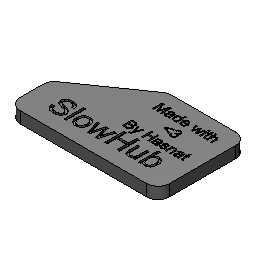
slowhub assembled (Autodesk Fusion 360 archive; units mm, degrees)
design "Slowhub Top"
part number: 2026-06-01-11-18-53-396
Autodesk Fusion 360 part; units mm, degrees
sketch "Sketch1" plane through (0, 0, 0) normal (0, 0, 1) x (1, 0, 0)
  arc A0 through (105.9986, -116.1185, 3) (107.7559, -120.3611, 3) (111.9985, -122.1184, 3)
  arc A1 through (177.7077, -122.1184, 3) (181.9503, -120.3611, 3) (183.7076, -116.1185, 3)
  arc A2 through (183.7076, -81.7289, 3) (181.9503, -77.4863, 3) (177.7077, -75.729, 3)
  arc A3 through (180.7076, -81.7289, 3) (179.829, -79.6076, 3) (177.7077, -78.729, 3)
  arc A4 through (144.4062, -75.729, 3) (142.6026, -76.0065, 3) (140.9659, -76.8133, 3)
  arc A5 through (108.5627, -99.4849, 3) (106.6768, -101.6374, 3) (106.0025, -104.4186, 3)
  arc A6 through (177.7077, -119.1184, 3) (179.829, -118.2398, 3) (180.7076, -116.1185, 3)
  arc A7 through (180.7076, -81.7289, 3) (179.829, -79.6076, 3) (177.7077, -78.729, 3)
  arc A8 through (144.4062, -78.729, 3) (143.5042, -78.8678, 3) (142.6857, -79.2713, 3)
  arc A9 through (110.2827, -101.9429, 3) (109.3377, -103.023, 3) (109.0025, -104.4186, 3)
  arc A10 through (108.9986, -116.1185, 3) (109.8772, -118.2398, 3) (111.9985, -119.1184, 3)
  line L0 (177.7077, -122.1184, 3) -> (111.9985, -122.1184, 3)
  line L1 (183.7076, -81.7289, 3) -> (183.7076, -116.1185, 3)
  line L2 (177.7077, -75.729, 3) -> (144.4062, -75.729, 3)
  line L3 (140.9659, -76.8133, 3) -> (108.5627, -99.4849, 3)
  line L4 (106.0025, -104.4186, 3) -> (105.9986, -116.1185, 3)
  line L5 (108.9986, -116.1185, 3) -> (109.0025, -104.4186, 3)
  line L6 (111.9985, -119.1184, 3) -> (177.7077, -119.1184, 3)
  line L7 (180.7076, -116.1185, 3) -> (180.7076, -81.7289, 3)
  line L8 (144.4062, -78.729, 3) -> (177.7077, -78.729, 3)
  line L9 (110.2827, -101.9429, 3) -> (142.6857, -79.2713, 3)
  point P0 (111.9985, -116.1185)
  point P1 (177.7077, -116.1185)
extrude "Extrude1" add sketch "Sketch1" along normal blind 3 contours A0 A1 A2 A4 A5 L0 L1 L2 L3 L4 | A3 A6 A7 A8 A9 A10 L5 L6 L7 L8 L9 in plane through (0, 0, 3) normal (0, 0, 1)
extrude "Extrude2" add sketch "Sketch1" against normal blind 3 contours A0 A1 A2 A4 A5 L0 L1 L2 L3 L4 in plane through (0, 0, 3) normal (0, 0, 1)
sketch "Sketch2" plane through (0, 0, 0) normal (0, 0, -1) x (1, 0, 0)
  arc A0 (111.9985, 119.1184) -> (108.9986, 116.1185) centre (111.9985, 116.1185) ccw
  line L0 (111.9985, 119.1184) -> (177.7077, 119.1184)
  arc A1 (180.7076, 116.1185) -> (177.7077, 119.1184) centre (177.7077, 116.1185) ccw
  line L1 (180.7076, 116.1185) -> (180.7076, 81.7289)
  arc A2 (177.7077, 78.729) -> (180.7076, 81.7289) centre (177.7077, 81.7289) ccw
  line L2 (177.7077, 78.729) -> (144.4062, 78.729)
  arc A3 (142.6857, 79.2713) -> (144.4062, 78.729) centre (144.4062, 81.729) ccw
  line L3 (142.6857, 79.2713) -> (110.2827, 101.9429)
  arc A4 (109.0025, 104.4186) -> (110.2827, 101.9429) centre (112.0024, 104.401) ccw
  line L4 (109.0025, 104.4186) -> (108.9986, 116.1185)
  arc A5 (177.7077, 75.729) -> (183.7076, 81.7289) centre (177.7077, 81.7289) ccw
  line L5 (183.7076, 81.7289) -> (183.7076, 116.1185)
  arc A6 (183.7076, 116.1185) -> (177.7077, 122.1184) centre (177.7077, 116.1185) ccw
  line L6 (177.7077, 122.1184) -> (111.9985, 122.1184)
  arc A7 (111.9985, 122.1184) -> (105.9986, 116.1185) centre (111.9985, 116.1185) ccw
  line L7 (105.9986, 116.1185) -> (106.0025, 104.4186)
  arc A8 (106.0025, 104.4186) -> (108.5627, 99.4849) centre (112.0024, 104.401) ccw
  line L8 (108.5627, 99.4849) -> (140.9659, 76.8133)
  arc A9 (140.9659, 76.8133) -> (144.4062, 75.729) centre (144.4062, 81.729) ccw
  line L9 (144.4062, 75.729) -> (177.7077, 75.729)
  line L10 (144.4062, 78.729) -> (177.7077, 78.729)
  line L11 (177.7077, 78.729) -> (177.7077, 77.229)
  line L12 (177.7077, 77.229) -> (144.4062, 77.229)
  line L13 (144.4062, 77.229) -> (144.4062, 78.729)
  line L14 (111.9985, 119.1184) -> (177.7077, 119.1184)
  line L15 (177.7077, 119.1184) -> (177.7077, 120.6184)
  line L16 (177.7077, 120.6184) -> (111.9985, 120.6184)
  line L17 (111.9985, 120.6184) -> (111.9985, 119.1184)
  dimension "d5" = 1.5
  dimension "d6" = 1.5
  constraint horizontal L10
  constraint vertical L11
  constraint horizontal L12
  constraint vertical L13
  constraint coincident L2.end A3.end
  constraint horizontal L14
  constraint vertical L15
  constraint horizontal L16
  constraint vertical L17
  constraint coincident A0.start L0.start
  measures "d5" distance of L2.end L12.end
  measures "d6" distance of A0.start L16.end
extrude "Extrude3" cut sketch "Sketch2" against normal blind 3 contours L0 L14 L15 L16 L17 | L2 L10 L11 L12 L13
fillet "Fillet1" radius 1.5 1 edges at (111.9985, -119.1184, 1.5)
fillet "Fillet2" radius 1.5 1 edges at (177.7077, -119.1184, 1.5)
fillet "Fillet3" radius 1.5 1 edges at (144.4062, -78.729, 1.5)
fillet "Fillet4" radius 1.5 1 edges at (177.7077, -78.729, 1.5)
chamfer "Chamfer1" distance 0.5 angle 45 1 edges at (161.0569, -77.229, 0)
chamfer "Chamfer2" distance 0.5 angle 45 1 edges at (144.8531, -120.6184, 0)
sketch "Sketch3" plane through (0, -77.229, 0) normal (0, -1, 0) x (1, 0, 0)
  line L0 (144.4062, 0.5) -> (177.7077, 0.5)
  line L1 (177.7077, 0.5) -> (177.7077, 3)
  line L2 (177.7077, 3) -> (144.4062, 3)
  line L3 (144.4062, 3) -> (144.4062, 0.5)
  line L4 (177.7077, 3) -> (144.4062, 3)
  line L5 (144.4062, 3) -> (144.4062, 1.5)
  line L6 (144.4062, 1.5) -> (177.7077, 1.5)
  line L7 (177.7077, 1.5) -> (177.7077, 3)
  dimension "d19" = 1.5
  constraint horizontal L4
  constraint vertical L5
  constraint horizontal L6
  constraint vertical L7
  constraint coincident L1.end L2.start
  measures "d19" distance of L1.end L6.end
extrude "Extrude4" cut sketch "Sketch3" against normal blind 6.369 draft -45 contours L1 L2 L3 L4 L5 L6 L7
fillet "Fillet5" radius 0.3 1 edges at (161.0569, -77.229, 1.5)
sketch "Sketch4" plane through (0, -120.6184, 0) normal (0, 1, 0) x (-1, 0, 0)
  line L0 (-177.7077, 0.5) -> (-111.9985, 0.5)
  line L1 (-111.9985, 0.5) -> (-111.9985, 3)
  line L2 (-111.9985, 3) -> (-177.7077, 3)
  line L3 (-177.7077, 3) -> (-177.7077, 0.5)
  line L4 (-111.9985, 3) -> (-177.7077, 3)
  line L5 (-177.7077, 3) -> (-177.7077, 1.5)
  line L6 (-177.7077, 1.5) -> (-111.9985, 1.5)
  line L7 (-111.9985, 1.5) -> (-111.9985, 3)
  dimension "d24" = 1.5
  constraint horizontal L4
  constraint vertical L5
  constraint horizontal L6
  constraint vertical L7
  constraint coincident L3 L5.end
  constraint coincident L1.end L2.start
  measures "d24" distance of L1.end L6.end
extrude "Extrude5" cut sketch "Sketch4" against normal blind 4 draft -45 contours L1 L2 L3 L4 L5 L6 L7
fillet "Fillet6" radius 0.3 1 edges at (144.8531, -120.6184, 1.5)
sketch "Sketch5" plane through (0, 0, 6) normal (0, 0, 1) x (-1, 0, 0)
  arc A0 (-183.7076, 81.7289) -> (-177.7077, 75.729) centre (-177.7077, 81.7289) ccw
  line L0 (-177.7077, 75.729) -> (-144.4062, 75.729)
  arc A1 (-144.4062, 75.729) -> (-140.9659, 76.8133) centre (-144.4062, 81.729) ccw
  line L1 (-140.9659, 76.8133) -> (-108.5627, 99.4849)
  arc A2 (-108.5627, 99.4849) -> (-106.0025, 104.4186) centre (-112.0024, 104.401) ccw
  line L2 (-106.0025, 104.4186) -> (-105.9986, 116.1185)
  arc A3 (-105.9986, 116.1185) -> (-111.9985, 122.1184) centre (-111.9985, 116.1185) ccw
  line L3 (-111.9985, 122.1184) -> (-177.7077, 122.1184)
  arc A4 (-177.7077, 122.1184) -> (-183.7076, 116.1185) centre (-177.7077, 116.1185) ccw
  line L4 (-183.7076, 116.1185) -> (-183.7076, 81.7289)
  line L5 (-112.0024, 116.1185) -> (-177.7077, 116.1185) construction
  line L6 (-177.7077, 116.1185) -> (-177.7077, 104.401) construction
  line L7 (-177.7077, 104.401) -> (-112.0024, 104.401) construction
  line L8 (-112.0024, 104.401) -> (-112.0024, 116.1185) construction
  line L9 (-144.4062, 104.401) -> (-177.7077, 104.401) construction
  line L10 (-177.7077, 104.401) -> (-177.7077, 81.729) construction
  line L11 (-177.7077, 81.729) -> (-144.4062, 81.729) construction
  line L12 (-144.4062, 81.729) -> (-144.4062, 104.401) construction
  dimension "d29" = 10
  dimension "d30" = 5
  text T0 "SlowHub" font "Arial" height 10 align centre top in box 65.7052 x 11.7174 at (-112.0024, 116.1185) x (-1, 0) y (0, -1) spacing 1 kerned
  text T1 "Made with <3\nBy Hasnat" font "Arial" height 5 align centre top in box 33.3015 x 22.6721 at (-144.4062, 104.401) x (-1, 0) y (0, -1) spacing 1 kerned
  constraint coincident A4.centre
  constraint coincident A2.centre
  constraint coincident A1.centre
extrude "Extrude6" cut sketch "Sketch5" against normal blind 1 text T1 T0
